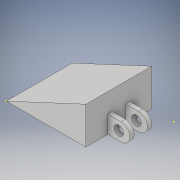
# Autodesk Inventor part: RoboArm 2020 scoop
Saved by Autodesk Inventor 2019 (Build 230136000, 136)
## iProperties
Created: 2020-02-03
Part Number: RoboArm 2020 scoop
Material: Generic
Document SubType Name: Modeling
Designer: mbird
Density: 1 g/cm^3
Appearance: Default
Author: mbird
Autodesk Inventor part; units mm, degrees
ref_plane "YZ Plane" through (0, 0, 0) normal (1, 0, 0) x (0, 1, 0)
ref_plane "XZ Plane" through (0, 0, 0) normal (0, 1, 0) x (-1, 0, 0)
ref_plane "XY Plane" through (0, 0, 0) normal (0, 0, 1) x (1, 0, 0)
sketch "Sketch1" plane through (0, 0, 0) normal (0, 0, 1) x (1, 0, 0)
  line L0 (0, 0) -> (181.2616, 84.5237)
  line L1 (0, 0) -> (200, 0) construction
  line L2 (0, 0) -> (181.2616, 0)
  line L3 (181.2616, 84.5237) -> (181.2616, 0)
  dimension "d2" = 200
  dimension "d3" = 25
  constraints: 8 end point, 1 equal length, 1 horizontal, 1 perpendicular, 1 point on line
  measures "d2" distance of L0.start L0.end
  measures "d3" angle of L1 L0
extrude "Extrusion1" add sketch "Sketch1" along normal blind 150
sketch "Sketch2" plane through (0, 0, 150) normal (0, 0, 1) x (1, 0, 0)
  point P0 (0, 0)
sketch "Sketch3" plane through (181.2616, 0, 0) normal (1, 0, 0) x (0, 0, -1)
  line L0 (-100, 0) -> (-50, 0)
  line L1 (-50, 0) -> (-50, 40)
  line L2 (-50, 40) -> (-100, 40)
  line L3 (-100, 40) -> (-100, 0)
  dimension "d10" = 50
  dimension "d11" = 40
  constraints: 8 end point, 2 parallel, 1 horizontal, 1 perpendicular
  measures "d10" distance of L2.end L1.end
  measures "d11" distance of L1.end L0.end
extrude "Extrusion2" add sketch "Sketch3" along normal blind 50
sketch "Sketch5" plane through (231.2616, 0, 0) normal (1, 0, 0) x (0, 0, -1)
  point P0 (0, 0)
sketch "Sketch6" plane through (231.2616, 0, 0) normal (1, 0, 0) x (0, 0, -1)
  line L0 (0, 0) -> (60, 0) construction
  line L1 (-60, 40) -> (-90, 40)
  line L2 (-90, 40) -> (-90, 0)
  line L3 (-90, 0) -> (-60, 0)
  line L4 (-60, 0) -> (-60, 40)
  dimension "d27" = 30
  dimension "d28" = 40
  constraints: 10 end point, 2 horizontal, 2 parallel, 1 perpendicular
  measures "d27" distance of L3.end L2.end
  measures "d28" distance of L2.end L1.end
extrude "Extrusion3" cut sketch "Sketch6" against normal blind 50
sketch "Sketch8" plane through (181.2616, 0, 100) normal (0, 0, 1) x (1, 0, 0)
  line L0 (50, 0) -> (50, 40) projected
  line L1 (0, 40) -> (0, 0) projected
  line L2 (0, 40) -> (50, 40) projected
  line L3 (0, 0) -> (50, 0) projected
  point P0 (-181.2616, 0)
  point P1 (25, 20)
hole "Hole2" at (206.2616, 20, 100) direction (0, 0, -1) diameter 22 end through all
fillet "Fillet1" radius 20 1 edges at (231.2616, 40, 95)
fillet "Fillet2" radius 20 1 edges at (231.2616, 0, 95)
fillet "Fillet3" radius 20 1 edges at (231.2616, 40, 55)
fillet "Fillet4" radius 20 1 edges at (231.2616, 0, 55)
body "Solid1"
